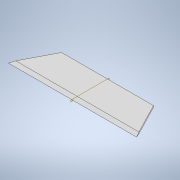
# Autodesk Inventor part: nóż
Saved by Autodesk Inventor 2022.3 (Build 263350000, 350)
## iProperties
Created: 2022-12-13
Part Number: nóż
Material: Generic
Document SubType Name: Modeling
Designer: komputer
Density: 1 g/cm^3
Appearance: Default
Author: komputer
Autodesk Inventor part; units mm, degrees
ref_plane "YZ Plane" through (0, 0, 0) normal (1, 0, 0) x (0, 1, 0)
ref_plane "XZ Plane" through (0, 0, 0) normal (0, 1, 0) x (-1, 0, 0)
ref_plane "XY Plane" through (0, 0, 0) normal (0, 0, 1) x (1, 0, 0)
sketch "Sketch1" plane through (0, 0, 0) normal (0, 1, 0) x (-1, 0, 0)
  line L0 (7.6807, 7.7641) -> (-42.3193, 7.7641)
  line L1 (7.6807, 7.7641) -> (-1.1191, -9.2324)
  line L2 (-17.3193, 7.7641) -> (-17.3193, -12.946)
  line L3 (-42.3193, 7.7641) -> (-33.5196, -9.2324)
  line L4 (-17.3193, -5.8724) -> (0.6205, -5.8724)
  line L5 (-35.2592, -5.8724) -> (-17.3193, -5.8724)
  point P0 (0, 0)
  dimension "d0" = 50
  constraints: 12 end point, 4 point on line, 2 horizontal, 1 collinear, 1 midpoint, 1 symmetric about line, 1 vertical
  measures "d0" distance of L0.start L0.end
extrude "Extrusion1" add sketch "Sketch1" along normal blind 0.6
ref_plane "Work Plane1" through (17.3193, 0, -40.5229) normal (-1, 0, 0) x (0, 1, 0)
sketch "Sketch2" plane through (17.3193, 0, -40.5229) normal (-1, 0, 0) x (0, 1, 0)
  line L0 (0, -48.2871) -> (0, -34.6505) projected
  line L1 (0, -34.6505) -> (0.6, -34.6505) projected
  line L2 (0.6, -48.2871) -> (0.6, -34.6505) projected
  line L3 (0, -48.2871) -> (0.6, -48.2871) projected
  line L4 (0.3, -48.2871) -> (0.6, -46.3953)
  line L5 (0.6, -34.6505) -> (0.6, -48.2871) projected
  line L6 (0.3, -48.2871) -> (0, -46.3953)
  line L7 (0, -34.6505) -> (0, -48.2871) projected
  point P0 (0, -40.5229)
  constraints: 4 end point, 2 point on line, 1 midpoint
extrude "Extrusion2" cut sketch "Sketch2" along normal mid plane 50 contours L0 L6 L3 | L4 L2 L3
body "Solid1"
